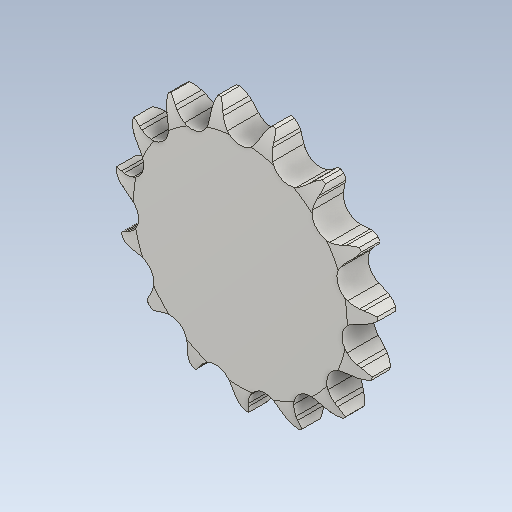
# Autodesk Inventor part: Rueda dentada de cadena de rodillos1
Saved by Autodesk Inventor 2020 (Build 240168000, 168)
## iProperties
Created: 2021-01-16
Part Number: Rueda dentada de cadena de rodillos1
Material: Steel
Document SubType Name: Modeling
Designer: pc-home
Density: 1 g/cm^3
Appearance: Steel
CustomPartVersion: 1
Author: pc-home
Autodesk Inventor part; units mm, degrees
ref_plane "YZ Plane" through (0, 0, 0) normal (1, 0, 0) x (0, 1, 0)
ref_plane "XZ Plane" through (0, 0, 0) normal (0, 1, 0) x (-1, 0, 0)
sketch "Perfil de diente teórico" plane through (0, 0, 0) normal (0, 0, 1) x (1, 0, 0)
  circle A0 centre (0, 0) radius 91.6254 construction
  line L0 (0, 0) -> (0, 91.6254) construction
  line L1 (0, 0) -> (37.2674, 83.704) construction
  circle A1 centre (0, 0) radius 101.0532
  arc A2 (-9.9685, 83.5531) -> (9.9685, 83.5531) centre (0, 91.6254) ccw
  line L2 (0, 91.6254) -> (37.2674, 83.704) construction
  line L3 (0, 91.6254) -> (15.7916, 104.4132) construction
  line L4 (15.7916, 104.4132) -> (-14.3147, 90.5447) construction
  arc A3 (19.6499, 99.1243) -> (15.4989, 93.1154) centre (34.7829, 84.2321) ccw
  arc A4 (-15.4989, 93.1154) -> (-19.6499, 99.1243) centre (-34.7829, 84.2321) ccw
  line L5 (-34.7829, 84.2321) -> (-15.4989, 93.1154) construction
  arc A5 (-14.3147, 90.5447) -> (-9.9685, 83.5531) centre (15.7916, 104.4132) ccw
  line L6 (-14.3147, 90.5447) -> (-15.4989, 93.1154)
  arc A6 (9.9685, 83.5531) -> (14.3147, 90.5447) centre (-15.7916, 104.4132) ccw
  line L7 (15.4989, 93.1154) -> (14.3147, 90.5447)
  line L8 (0, 0) -> (21.0101, 98.8449) construction
  point P0 (18.6337, 87.6647)
  dimension "d0" = 183.2509
  dimension "d2" = 24
  dimension "d3" = 12.827
  dimension "d10" = 129
  dimension "d11" = 14.267
  dimension "d12" = 20.32
  dimension "d13" = 33.147
  dimension "d14" = 35.56
  dimension "d23" = 11.43
  constraints: 18 end point, 15 point on circle, 7 centre point, 3 coincident, 3 point on line, 3 symmetric about line, 3 tangent, 1 equal radius, 1 midpoint, 1 parallel, 1 vertical, 1 other
  measures "d0" diameter of A0
  measures "d2" angle of L1 L0
  measures "d3" radius of A2
  measures "d10" angle of L3 L0
  measures "d11" angle of L4 L3
  measures "d12" distance of L2.start L3.end
  measures "d13" distance of L3.end L4.end
  measures "d14" distance of A3.centre L0.end
  measures "d23" distance from line of L8.end L2
sketch "Perfil de diente" plane through (0, 0, 0) normal (0, 0, 1) x (1, 0, 0)
  arc A0 (-11.8073, 86.6135) -> (11.8073, 86.6135) centre (0, 91.6254) ccw
  arc A1 (19.3967, 99.1742) -> (11.8073, 86.6135) centre (59.5042, 66.3674) ccw
  arc A2 (-11.8073, 86.6135) -> (-19.3967, 99.1742) centre (-59.5042, 66.3674) ccw
  line L0 (0, 0) -> (0, 91.6254) construction
  line L1 (0, 91.6254) -> (11.8073, 86.6135) construction
  line L2 (0, 91.6254) -> (-11.8073, 86.6135) construction
  circle A3 centre (0, 0) radius 101.0532 projected
  dimension "d44" = 134
  dimension "d45" = 51.816
  dimension "d46" = 12.827
  constraints: 9 point on circle, 6 end point, 3 centre point, 2 tangent, 1 coincident, 1 equal radius, 1 vertical, 1 other
  measures "d44" angle of L2 L1
  measures "d45" radius of A1
  measures "d46" radius of A0
sketch "Perfil de sección" plane through (0, 0, 0) normal (1, 0, 0) x (0, 1, 0)
  line L0 (101.0532, 0) -> (-101.0532, 0) projected
  line L1 (66.9312, 12.065) -> (-66.9312, 12.065)
  line L2 (-66.9312, 12.065) -> (-66.9312, -12.065)
  line L3 (-66.9312, -12.065) -> (66.9312, -12.065)
  line L4 (66.9312, -12.065) -> (66.9312, 12.065)
  line L5 (66.9312, 12.065) -> (101.0532, 12.065) construction
  line L6 (101.0532, 12.065) -> (101.0532, -12.065) construction
  line L7 (101.0532, -12.065) -> (66.9312, -12.065) construction
  line L8 (66.9312, -12.065) -> (66.9312, 12.065)
  arc A0 (101.0532, 7.112) -> (82.2679, 12.065) centre (82.2679, -26.035) ccw
  arc A1 (82.2679, -12.065) -> (101.0532, -7.112) centre (82.2679, 26.035) ccw
  line L9 (82.2679, 12.065) -> (0, 12.065)
  line L10 (0, 12.065) -> (0, -12.065)
  line L11 (0, -12.065) -> (82.2679, -12.065)
  line L12 (0, 12.065) -> (0, -12.065)
  line L13 (101.0532, 7.112) -> (101.0532, -7.112)
  point P0 (0, 0)
  point P1 (0, 0)
  dimension "d30" = 24.13
  dimension "d31" = 133.8624
  dimension "d32" = 24.13
  dimension "d33" = 4.953
  dimension "d34" = 38.1
  dimension "d43" = 12.065
  constraints: 26 end point, 7 midpoint, 5 perpendicular, 4 parallel, 4 point on circle, 3 point on line, 3 symmetric about line, 2 centre point, 2 horizontal, 2 tangent, 1 collinear, 1 other
  measures "d30" distance between parallel lines of L7 L5
  measures "d31" distance between parallel lines of L2 L4
  measures "d32" distance between parallel lines of L3 L1
  measures "d33" distance from line of L13.start L5
  measures "d34" radius of A0
  measures "d43" distance between parallel lines of L3 L0
revolve "Cubierta" add sketch "Perfil de sección" angle 360 about axis through (0, 0, 12.065) along (0, 0, -1) contours L10 L3 L2 L0 | L0 L2 L1 L10
revolve "Ramal" add sketch "Perfil de sección" angle 360 about axis through (0, 0, 12.065) along (0, 0, -1) contours L13 A1 L11 L4 L0 | L0 L4 L9 A0 L13 | L4 L3 L10 L0 | L0 L10 L1 L4
pattern_of_one "Patrón de ramal"
extrude "Diente teórico" cut sketch "Perfil de diente teórico" along normal through all both and the other way through all contours A3 L7 A6 A2 A5 L6 A4 A1 picked at (0, 93.4916)
extrude "Diente" [suppressed]
pattern_circular "Patrón de diente" count 15 over 360 about axis through (0, 0, -10) along (0, 0, 1) of "Diente teórico"
ref_plane "Plano síncrono" through (0, 91.6254, 0) normal (1, 0, 0) x (0, 1, 0)
equation "\"d3\" = 0.5 * da_Dr + da_SC"
equation "\"d12\" = 0.8 * da_Dr"
equation "\"d13\" = 1.3 * da_Dr + da_SC"
equation "\"d14\" = 1.4 * da_Dr"
equation "\"d23\" = da_Ha"
equation "\"d44\" = da_Alfa"
equation "\"d45\" = da_Re"
equation "\"d46\" = da_Ri"
equation "\"d30\" = da_Bf"
equation "\"d31\" = da_Ds"
equation "\"d32\" = da_Bs"
equation "\"d33\" = da_Ba"
equation "\"d34\" = da_Rx"
equation "\"d40\" = da_pt"
equation "\"form_type\" = 0"
equation "\"da_p\" = 38.1"
equation "\"da_Dr\" = 25.4"
equation "\"da_SC\" = 0.127"
equation "\"da_Ha\" = 11.43"
equation "\"da_pt\" = 48.36"
equation "\"da_Bf\" = 24.13"
equation "\"da_Ba\" = 4.953"
equation "\"da_Rx\" = 38.1"
equation "\"da_Ra\" = 1.524"
equation "\"da_Bs\" = 24.13"
equation "\"da_Ds\" = 133.86241"
equation "\"da_Re\" = 51.816"
equation "\"da_Ri\" = 12.827"
equation "\"da_Alfa\" = 134deg"
body "Solid1"
